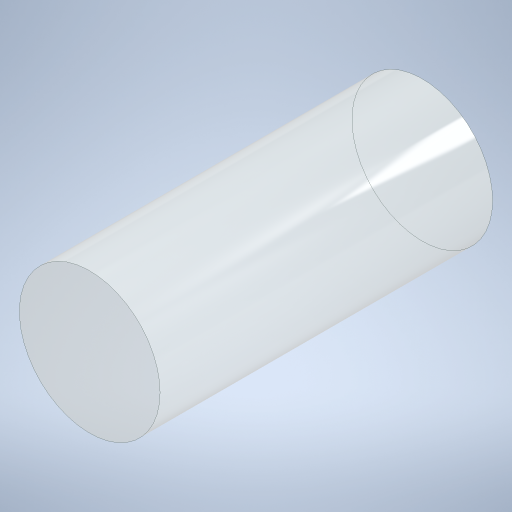
# Autodesk Inventor part: fuse_fuse
Saved by Autodesk Inventor 2024.1 (Build 281209000, 209)
## iProperties
Created: 2025-02-19
Part Number: fuse_fuse
Material: ガラス
Document SubType Name: Modeling
Designer: hibik
Density: 2.18 g/cm^3
Appearance: クリア
Author: hibik
Autodesk Inventor part; units mm, degrees
ref_plane "YZ Plane" through (0, 0, 0) normal (1, 0, 0) x (0, 1, 0)
ref_plane "XZ Plane" through (0, 0, 0) normal (0, 1, 0) x (-1, 0, 0)
ref_plane "XY Plane" through (0, 0, 0) normal (0, 0, 1) x (1, 0, 0)
sketch "スケッチ1" plane through (0, 0, 0) normal (0, 0, 1) x (1, 0, 0)
  circle A0 centre (0, 0) radius 2.75
  dimension "d0" = 5.5
  constraints: 1 centre point, 1 coincident
  measures "d0" diameter of A0
extrude "押し出し1" add sketch "スケッチ1" along normal blind 6.5
mirror "ミラー1" about plane through (0, 0, 0) normal (0, 0, -1)
